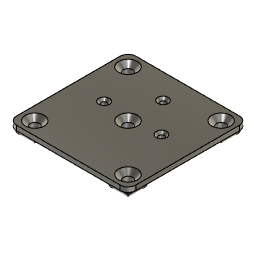
DIYbio orbital shaker bearing linkage (Autodesk Fusion 360 archive; units mm, degrees)
design "modifiedShakerPlatform v2"
Autodesk Fusion 360 part; units mm, degrees
mesh "Mesh2" [no effect]
mesh "Mesh3" [no effect]
sketch "Sketch2" plane through (0, 0, 0) normal (0, 0, 1) x (1, 0, 0)
  line L0 (-37.5, 37.5) -> (37.5, 37.5)
  line L1 (37.5, 37.5) -> (37.5, -37.5)
  line L2 (37.5, -37.5) -> (-37.5, -37.5)
  line L3 (-37.5, -37.5) -> (-37.5, 37.5)
  line L4 (-37.5, 37.5) -> (37.5, -37.5) construction
  line L5 (37.5, 37.5) -> (-37.5, -37.5) construction
  circle A0 centre (0, 22) radius 1.8
  circle A1 centre (-18, 3) radius 1.8
  circle A2 centre (18, 3) radius 1.8
  circle A3 centre (-29.25, 29.25) radius 2.9
  circle A4 centre (29.25, 29.25) radius 2.9
  circle A5 centre (-29.25, -29.25) radius 2.9
  circle A6 centre (29.25, -29.25) radius 2.9
  circle A7 centre (0, 0) radius 2.9
  line L6 (-7, 7) -> (7, 7)
  line L7 (7, 7) -> (7, -7)
  line L8 (7, -7) -> (-7, -7)
  line L9 (-7, -7) -> (-7, 7)
  line L10 (-7, 7) -> (7, -7) construction
  line L11 (7, 7) -> (-7, -7) construction
  line L12 (-35.25, 35.25) -> (-23.25, 35.25)
  line L13 (-23.25, 35.25) -> (-23.25, 23.25)
  line L14 (-23.25, 23.25) -> (-35.25, 23.25)
  line L15 (-35.25, 23.25) -> (-35.25, 35.25)
  line L16 (-35.25, 35.25) -> (-23.25, 23.25) construction
  line L17 (-23.25, 35.25) -> (-35.25, 23.25) construction
  line L18 (23.25, 35.25) -> (35.25, 35.25)
  line L19 (35.25, 35.25) -> (35.25, 23.25)
  line L20 (35.25, 23.25) -> (23.25, 23.25)
  line L21 (23.25, 23.25) -> (23.25, 35.25)
  line L22 (23.25, 35.25) -> (35.25, 23.25) construction
  line L23 (35.25, 35.25) -> (23.25, 23.25) construction
  line L24 (23.25, -23.25) -> (35.25, -23.25)
  line L25 (35.25, -23.25) -> (35.25, -35.25)
  line L26 (35.25, -35.25) -> (23.25, -35.25)
  line L27 (23.25, -35.25) -> (23.25, -23.25)
  line L28 (23.25, -23.25) -> (35.25, -35.25) construction
  line L29 (35.25, -23.25) -> (23.25, -35.25) construction
  line L30 (-23.25, -23.25) -> (-35.25, -23.25)
  line L31 (-35.25, -23.25) -> (-35.25, -35.25)
  line L32 (-35.25, -35.25) -> (-23.25, -35.25)
  line L33 (-23.25, -35.25) -> (-23.25, -23.25)
  line L34 (-23.25, -23.25) -> (-35.25, -35.25) construction
  line L35 (-35.25, -23.25) -> (-23.25, -35.25) construction
  line L36 (-21, 0) -> (-15, 0)
  line L37 (-15, 0) -> (-15, 6)
  line L38 (-15, 6) -> (-21, 6)
  line L39 (-21, 6) -> (-21, 0)
  line L40 (-21, 0) -> (-15, 6) construction
  line L41 (-15, 0) -> (-21, 6) construction
  line L42 (21, 0) -> (15, 0)
  line L43 (15, 0) -> (15, 6)
  line L44 (15, 6) -> (21, 6)
  line L45 (21, 6) -> (21, 0)
  line L46 (21, 0) -> (15, 6) construction
  line L47 (15, 0) -> (21, 6) construction
  line L48 (-3, 19) -> (3, 19)
  line L49 (3, 19) -> (3, 25)
  line L50 (3, 25) -> (-3, 25)
  line L51 (-3, 25) -> (-3, 19)
  line L52 (-3, 19) -> (3, 25) construction
  line L53 (3, 19) -> (-3, 25) construction
  point P0 (-29.25, 29.25)
  point P1 (29.25, 29.25)
  point P2 (29.25, -29.25)
  point P3 (-29.25, -29.25)
  point P4 (-18, 3)
  point P5 (18, 3)
  point P6 (0, 22)
  dimension "d5" = 75
  dimension "d6" = 75
  dimension "d7" = 3.6
  dimension "d8" = 3.6
  dimension "d9" = 3.6
  dimension "d10" = 19.5
  dimension "d11" = 19.5
  dimension "d12" = 37.5
  dimension "d13" = 37.5
  dimension "d14" = 34.5
  dimension "d15" = 34.5
  dimension "d16" = 5.8
  dimension "d17" = 8.25
  dimension "d18" = 8.25
  dimension "d19" = 5.8
  dimension "d20" = 8.25
  dimension "d21" = 8.25
  dimension "d22" = 59
  dimension "d23" = 5.8
  dimension "d24" = 5.8
  dimension "d25" = 8.25
  dimension "d26" = 8.25
  dimension "d27" = 8.25
  dimension "d28" = 8.25
  dimension "d29" = 61.5
  dimension "d34" = 5.8
  dimension "d37" = 14
  dimension "d38" = 12
  dimension "d39" = 12
  dimension "d40" = 12
  dimension "d41" = 12
  dimension "d42" = 12
  dimension "d43" = 12
  dimension "d44" = 12
  dimension "d45" = 12
  dimension "d50" = 6
  dimension "d51" = 6
  dimension "d52" = 6
  dimension "d53" = 6
  dimension "d54" = 6
  dimension "d55" = 6
  dimension "d58" = 36
  dimension "d59" = 19.5
  dimension "d60" = 18
  dimension "d61" = 20
  dimension "d62" = 19
  dimension "d63" = 37.5
  dimension "d64" = 39.5816
  constraint perpendicular L0 L1
  constraint parallel L0 L2
  constraint parallel L1 L3
  constraint horizontal L0
  constraint coincident L4 A7.centre
  constraint coincident L5 A7.centre
  constraint coincident A7.centre origin
  constraint perpendicular L6 L7
  constraint parallel L6 L8
  constraint parallel L7 L9
  constraint horizontal L6
  constraint coincident L10 A7.centre
  constraint coincident L11 A7.centre
  constraint perpendicular L12 L13
  constraint parallel L12 L14
  constraint parallel L13 L15
  constraint horizontal L12
  constraint coincident L16 P0
  constraint coincident L17 P0
  constraint coincident P0 A3.centre
  constraint perpendicular L18 L19
  constraint parallel L18 L20
  constraint parallel L19 L21
  constraint horizontal L18
  constraint coincident L22 P1
  constraint coincident L23 P1
  constraint coincident P1 A4.centre
  constraint perpendicular L24 L25
  constraint parallel L24 L26
  constraint parallel L25 L27
  constraint horizontal L24
  constraint coincident L28 P2
  constraint coincident L29 P2
  constraint coincident P2 A6.centre
  constraint perpendicular L30 L31
  constraint parallel L30 L32
  constraint parallel L31 L33
  constraint horizontal L30
  constraint coincident L34 P3
  constraint coincident L35 P3
  constraint coincident P3 A5.centre
  constraint perpendicular L36 L37
  constraint parallel L36 L38
  constraint parallel L37 L39
  constraint horizontal L36
  constraint coincident L40 P4
  constraint coincident L41 P4
  constraint coincident P4 A1.centre
  constraint perpendicular L42 L43
  constraint parallel L42 L44
  constraint parallel L43 L45
  constraint horizontal L42
  constraint coincident L46 P5
  constraint coincident L47 P5
  constraint coincident P5 A2.centre
  constraint perpendicular L48 L49
  constraint parallel L48 L50
  constraint parallel L49 L51
  constraint horizontal L48
  constraint coincident L52 P6
  constraint coincident L53 P6
  constraint coincident A0.centre P6
  measures "d5" distance of L0.end L1.end
  measures "d6" distance of L1.end L2.end
  measures "d7" diameter of A0
  measures "d8" diameter of A1
  measures "d9" diameter of A2
  measures "d10" distance of L3 P4
  measures "d11" distance of L1 P5
  measures "d12" distance of L1 A0.centre
  measures "d13" distance of L3 A0.centre
  measures "d14" distance of L0 P5
  measures "d15" distance of L0 P4
  measures "d16" diameter of A3
  measures "d17" distance of L3 P0
  measures "d18" distance of L0 P0
  measures "d19" diameter of A4
  measures "d20" distance of L0 P1
  measures "d21" distance of L1 P1
  measures "d23" diameter of A5
  measures "d24" diameter of A6
  measures "d25" distance of L1 P2
  measures "d26" distance of L3 P3
  measures "d27" distance of L2 P3
  measures "d28" distance of L2 P2
  measures "d34" diameter of A7
  measures "d37" distance of L6.end L7.end
  measures "d38" distance of L13.end L14.end
  measures "d39" distance of L12.end L13.end
  measures "d40" distance of L19.end L20.end
  measures "d41" distance of L18.end L19.end
  measures "d42" distance of L25.end L26.end
  measures "d43" distance of L24.end L25.end
  measures "d44" distance of L30.end L31.end
  measures "d45" distance of L31.end L32.end
  measures "d50" distance of L37.end L38.end
  measures "d51" distance of L36.end L37.end
  measures "d52" distance of L43.end L44.end
  measures "d53" distance of L42.end L43.end
  measures "d54" distance of L49.end L50.end
  measures "d55" distance of L48.end L49.end
  measures "d58" distance of P4 P5
  measures "d59" distance of L3 P4
  measures "d60" horizontal distance of A7.centre P4
  measures "d62" vertical distance of A0.centre P5
  measures "d63" distance of L2 A7.centre
extrude "Extrude2" add sketch "Sketch2" along normal blind 3 contours L0 L1 L2 L3 | L6 L7 L8 L9 | L12 L13 L14 L15 | L18 L19 L20 L21 | L24 L25 L26 L27 | L30 L31 L32 L33 | L36 L37 L38 L39 | L42 L43 L44 L45 | L48 L49 L50 L51
extrude "Extrude3" add sketch "Sketch2" against normal blind 5 contours L6 L7 L8 L9 | L12 L13 L14 L15 | L18 L19 L20 L21 | L24 L25 L26 L27 | L30 L31 L32 L33
extrude "Extrude4" add sketch "Sketch2" against normal blind 5 contours L36 L37 L38 L39 | L42 L43 L44 L45 | L48 L49 L50 L51
fillet "Fillet1" radius 5 4 edges at (-37.5, -37.5, 1.5) (37.5, -37.5, 1.5) (37.5, 37.5, 1.5) (-37.5, 37.5, 1.5)
chamfer "Chamfer2" distance 3 angle 45 5 edges at (-31.9537, 30.2987, 3) (26.5463, 30.2987, 3) (-2.7037, 1.0487, 3) (-31.9537, -28.2013, 3) (26.5463, -28.2013, 3)
chamfer "Chamfer3" distance 1.5 angle 45 3 edges at (-1.6782, 22.6509, 3) (-19.6782, 3.6509, 3) (16.3218, 3.6509, 3)
fillet "Fillet3" radius 3 20 edges at (29.25, -23.25, -5) (23.25, -29.25, -5) (29.25, -35.25, -5) (35.25, -29.25, -5) (35.25, 29.25, -5) (29.25, 35.25, -5) (23.25, 29.25, -5) (29.25, 23.25, -5) (-23.25, -29.25, -5) (-29.25, -23.25, -5) (-35.25, -29.25, -5) (-29.25, -35.25, -5) (-23.25, 29.25, -5) (-29.25, 35.25, -5) (-35.25, 29.25, -5) (-29.25, 23.25, -5) (0, 7, -5) (-7, 0, -5) (0, -7, -5) (7, 0, -5)
named bodies: "flask shaker platform"
